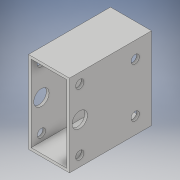
# Autodesk Inventor part: back support bearing holder
Saved by Autodesk Inventor 2018 (Build 220112000, 112)
## iProperties
Created: 2019-03-20
Part Number: back support bearing holder
Material: Generic
Document SubType Name: Modeling
Designer: S-4008082
Density: 1 g/cm^3
Appearance: Default
Author: S-4008082
Autodesk Inventor part; units mm, degrees
ref_plane "YZ Plane" through (0, 0, 0) normal (1, 0, 0) x (0, 1, 0)
ref_plane "XZ Plane" through (0, 0, 0) normal (0, 1, 0) x (-1, 0, 0)
ref_plane "XY Plane" through (0, 0, 0) normal (0, 0, 1) x (1, 0, 0)
sketch "Sketch1" plane through (0, 0, 0) normal (0, 0, 1) x (1, 0, 0)
  line L0 (12.7, -25.4) -> (-12.7, -25.4)
  line L1 (-12.7, -25.4) -> (-12.7, 25.4)
  line L2 (-12.7, 25.4) -> (12.7, 25.4)
  line L3 (12.7, 25.4) -> (12.7, -25.4)
  line L4 (11.049, -23.749) -> (-11.049, -23.749)
  line L5 (-11.049, -23.749) -> (-11.049, 23.749)
  line L6 (-11.049, 23.749) -> (11.049, 23.749)
  line L7 (11.049, 23.749) -> (11.049, -23.749)
  dimension "d0" = 25.4
  dimension "d1" = 50.8
  dimension "d2" = 1.651
  dimension "d3" = 1.651
  dimension "d4" = 1.651
  dimension "d5" = 1.651
  constraints: 16 end point, 4 parallel, 2 horizontal, 2 perpendicular
  measures "d0" distance of L1.end L2.end
  measures "d1" distance of L2.end L0.start
  measures "d2" distance between parallel lines of L2 L6
  measures "d3" distance between parallel lines of L3 L7
  measures "d4" distance between parallel lines of L4 L0
  measures "d5" distance between parallel lines of L1 L5
extrude "Extrusion1" add sketch "Sketch1" along normal blind 50.8
sketch "Sketch2" plane through (12.7, -25.4, 0) normal (1, 0, 0) x (0, 0, -1)
  circle A0 centre (-44.45, 25.4) radius 4.7625
  line L0 (-50.8, 0) -> (-50.8, 50.8) projected
  line L1 (0, 0) -> (-50.8, 0) projected
  point P0 (0, 25.4)
  dimension "d8" = 9.525
  dimension "d9" = 6.35
  dimension "d10" = 25.4
  constraints: 1 centre point
  measures "d8" diameter of A0
  measures "d9" distance from line of L0 A0.centre
  measures "d10" distance from line of L1 A0.centre
extrude "Extrusion2" cut sketch "Sketch2" against normal blind 50.8
sketch "Sketch3" plane through (12.7, -25.4, 0) normal (1, 0, 0) x (0, 0, -1)
  circle A0 centre (-10.16, 10.16) radius 2.5797
  circle A1 centre (-44.45, 6.35) radius 2.5797
  circle A2 centre (-44.45, 44.45) radius 2.5797
  circle A3 centre (-10.16, 40.64) radius 2.5797
  line L0 (0, 50.8) -> (-50.8, 50.8) projected
  line L1 (0, 50.8) -> (0, 0) projected
  line L2 (0, 0) -> (-50.8, 0) projected
  line L3 (-50.8, 0) -> (-50.8, 50.8) projected
  point P0 (0, 25.4)
  dimension "d13" = 10.16
  dimension "d14" = 10.16
  dimension "d15" = 6.35
  dimension "d16" = 6.35
  dimension "d17" = 6.35
  dimension "d18" = 6.35
  dimension "d19" = 10.16
  dimension "d20" = 10.16
  dimension "d21" = 5.1594
  dimension "d22" = 5.1594
  dimension "d23" = 5.1594
  dimension "d24" = 5.1594
  constraints: 4 centre point
  measures "d13" distance from line of L0 A3.centre
  measures "d14" distance from line of L1 A3.centre
  measures "d15" distance from line of L0 A2.centre
  measures "d16" distance from line of L2 A1.centre
  measures "d17" distance from line of L3 A1.centre
  measures "d18" distance from line of L3 A2.centre
  measures "d19" distance from line of L2 A0.centre
  measures "d20" distance from line of L1 A0.centre
  measures "d21" diameter of A0
  measures "d22" diameter of A3
  measures "d23" diameter of A1
  measures "d24" diameter of A2
extrude "Extrusion3" cut sketch "Sketch3" against normal blind 50.8 contours A0 | A1 | A2 | A3
equation "\"d3\" = d2"
equation "\"d5\" = d3"
equation "\"d14\" = d13"
equation "\"d16\" = d15"
equation "\"d17\" = d15"
equation "\"d18\" = d15"
equation "\"d19\" = d13"
equation "\"d20\" = d13"
equation "\"d22\" = d21"
equation "\"d23\" = d21"
equation "\"d24\" = d21"
body "Solid1"
